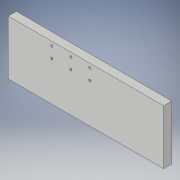
# Autodesk Inventor part: Short Plank
Saved by Autodesk Inventor 2018 (Build 220112000, 112)
## iProperties
Created: 2020-01-22
Part Number: Short Plank
Material: Generic
Document SubType Name: Modeling
Designer: s-2512711
Density: 1 g/cm^3
Appearance: Default
Author: s-2512711
Autodesk Inventor part; units mm, degrees
ref_plane "YZ Plane" through (0, 0, 0) normal (1, 0, 0) x (0, 1, 0)
ref_plane "XZ Plane" through (0, 0, 0) normal (0, 1, 0) x (-1, 0, 0)
ref_plane "XY Plane" through (0, 0, 0) normal (0, 0, 1) x (1, 0, 0)
sketch "Sketch1" plane through (0, 0, 0) normal (0, 0, 1) x (1, 0, 0)
  line L0 (0, 0) -> (361.95, 0)
  line L1 (361.95, 0) -> (361.95, 127)
  line L2 (361.95, 127) -> (0, 127)
  line L3 (0, 127) -> (0, 0)
  dimension "d0" = 361.95
  dimension "d1" = 127
  constraints: 8 end point, 2 parallel, 1 horizontal, 1 perpendicular
  measures "d0" distance of L2.end L1.end
  measures "d1" distance of L1.end L0.end
extrude "Extrusion1" add sketch "Sketch1" along normal blind 19.05
sketch "Sketch2" plane through (0, 0, 19.05) normal (0, 0, 1) x (1, 0, 0)
  line L0 (361.95, 127) -> (0, 127) construction
  line L1 (0, 127) -> (101.6, 127) construction
  line L2 (101.6, 127) -> (101.6, 117.475) construction
  line L3 (101.6, 117.475) -> (146.05, 117.475) construction
  line L4 (146.05, 117.475) -> (190.5, 117.475) construction
  line L5 (190.5, 117.475) -> (190.5, 92.075) construction
  line L6 (190.5, 92.075) -> (146.05, 92.075) construction
  line L7 (146.05, 92.075) -> (101.6, 92.075) construction
  circle A0 centre (101.6, 117.475) radius 2.667
  circle A1 centre (146.05, 117.475) radius 2.667
  circle A2 centre (190.5, 117.475) radius 2.667
  circle A3 centre (190.5, 92.075) radius 2.667
  circle A4 centre (146.05, 92.075) radius 2.667
  circle A5 centre (101.6, 92.075) radius 2.667
  point P0 (0, 0)
  dimension "d4" = 101.6
  dimension "d5" = 9.525
  dimension "d6" = 44.45
  dimension "d7" = 44.45
  dimension "d8" = 25.4
  dimension "d9" = 5.334
  constraints: 14 end point, 6 centre point, 6 coincident, 3 perpendicular, 3 point on line, 1 horizontal
  measures "d4" distance of L0.end L1.end
  measures "d5" distance of L1.end L2.end
  measures "d6" distance of L2.end L3.end
  measures "d7" distance of L3.end L4.end
  measures "d8" distance of L4.end L5.end
  measures "d9" diameter of A0
extrude "Extrusion2" cut sketch "Sketch2" against normal blind 19.05
body "Solid1"
